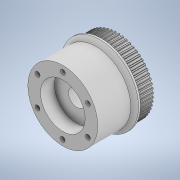
# Autodesk Inventor part: pulley_bearing_combo
Saved by Autodesk Inventor 2020.3 (Build 243373000, 373)
## iProperties
Created: 2020-11-01
Part Number: pulley_bearing_combo
Material: Generic
Document SubType Name: Modeling
Designer: Martijn
Density: 1 g/cm^3
Appearance: Default
Author: Martijn
Autodesk Inventor part; units mm, degrees
ref_plane "YZ Plane" through (0, 0, 0) normal (1, 0, 0) x (0, 1, 0)
ref_plane "XZ Plane" through (0, 0, 0) normal (0, 1, 0) x (-1, 0, 0)
ref_plane "XY Plane" through (0, 0, 0) normal (0, 0, 1) x (1, 0, 0)
sketch "Sketch1" plane through (0, 0, 0) normal (0, 0, 1) x (1, 0, 0)
  circle A0 centre (0, 0) radius 20
  circle A1 centre (0, 0) radius 11
  dimension "d0" = 40
  dimension "d1" = 22
  constraints: 2 centre point, 2 coincident
  measures "d0" diameter of A0
  measures "d1" diameter of A1
extrude "Extrusion1" add sketch "Sketch1" along normal blind 7
sketch "Sketch2" plane through (0, 0, 7) normal (0, 0, 1) x (1, 0, 0)
  circle A0 centre (0, 0) radius 4.3
  circle A1 centre (0, 0) radius 20
  circle A2 centre (0, 0) radius 20 projected
  dimension "d4" = 8.6
  constraints: 2 centre point, 2 coincident, 1 concentric
  measures "d4" diameter of A0
extrude "Extrusion2" add sketch "Sketch2" along normal blind 16
sketch "Sketch3" plane through (0, 0, 23) normal (0, 0, 1) x (1, 0, 0)
  circle A0 centre (0, 0) radius 90
  circle A1 centre (0, 0) radius 4.3
  circle A2 centre (0, 0) radius 4.3 projected
  dimension "d7" = 180
  constraints: 2 centre point, 2 coincident, 1 concentric
  measures "d7" diameter of A0
extrude "Extrusion3" add sketch "Sketch3" along normal blind 5
sketch "Sketch4" plane through (0, 0, 28) normal (0, 0, 1) x (1, 0, 0)
  circle A0 centre (0, 0) radius 20 projected
  circle A1 centre (0, 0) radius 11
  circle A2 centre (0, 0) radius 4.3 projected
  circle A3 centre (0, 0) radius 90
  circle A4 centre (0, 0) radius 90 projected
  dimension "d10" = 22
  constraints: 2 centre point, 2 coincident, 1 concentric
  measures "d10" diameter of A1
extrude "Extrusion4" add sketch "Sketch4" along normal blind 7 contours A0 | A3
sketch "Sketch5" plane through (0, 0, 0) normal (0, 0, -1) x (-1, 0, 0)
  circle A0 centre (0, 0) radius 20 projected
  line L0 (0, 0) -> (0, 20)
  arc A1 (-0.4919, 18.354) -> (0, 18.05) centre (0, 18.6) ccw
  circle A2 centre (0, 0) radius 4.3 projected
  arc A3 (-0.5869, 18.657) -> (-0.4919, 18.354) centre (0.4, 18.8) ccw
  line L1 (0.4, 18.8) -> (0, 18.8)
  line L2 (0, -98) -> (0, 98) projected
  arc A4 (-0.5869, 18.657) -> (-0.7413, 18.7854) centre (-0.7354, 18.6355) ccw
  line L3 (-1.0467, 19.9726) -> (0, 0)
  arc A5 (-0.7413, 18.7854) -> (-0.9839, 18.7742) centre (0, 0) ccw
  line L4 (-0.9839, 18.7742) -> (-1.0467, 19.9726)
  line L5 (0, 18.05) -> (0, 18.8)
  line L6 (0, 18.8) -> (0, 20)
  dimension "d14" = 0.55
  dimension "d17" = 0.4
  dimension "d18" = 0.75
  dimension "d19" = 0.15
  dimension "d20" = 3
  dimension "d22" = 18.8
  constraints: 12 end point, 10 point on circle, 5 point on line, 4 centre point, 4 collinear, 3 tangent, 1 coincident, 1 equal length, 1 perpendicular
  measures "d14" radius of A1
  measures "d17" distance of L1.start L1.end
  measures "d18" distance of L5.start L1.end
  measures "d19" radius of A4
  measures "d20" angle of L3 L0
  measures "d22" distance of L1.end L0.start
extrude "Extrusion5" cut sketch "Sketch5" against normal blind 8 contours L0 A1 A3 A4 A5 L3 A0
mirror "Mirror1" about plane through (0, 20, 0) normal (1, 0, 0) of "Extrusion5"
pattern_circular "Circular Pattern1" count 60 over 360 about axis through (0, 0, 7) along (0, 0, 1) of "Extrusion5", "Mirror1"
sketch "Sketch6" plane through (0, 0, 0) normal (0, 0, -1) x (-1, 0, 0)
  circle A0 centre (14, 0) radius 1.25
  line L0 (98, 0) -> (-98, 0) projected
  point P0 (0, 0)
  dimension "d28" = 2.5
  dimension "d29" = 14
  constraints: 1 centre point, 1 point on line
  measures "d28" diameter of A0
  measures "d29" distance of A0.centre point (0, 0)
extrude "Extrusion6" cut sketch "Sketch6" against normal blind 23
pattern_circular "Circular Pattern2" count 3 over 360 about axis through (0, 0, 7) along (0, 0, 1) of "Extrusion6"
sketch "Sketch7" plane through (0, 0, 28) normal (0, 0, 1) x (1, 0, 0)
  circle A0 centre (0, 0) radius 7.5
  dimension "d35" = 15
  constraints: 1 centre point, 1 coincident
  measures "d35" diameter of A0
extrude "Extrusion7" cut sketch "Sketch7" against normal blind 7.2
sketch "Sketch8" plane through (0, 0, 35) normal (0, 0, 1) x (1, 0, 0)
  circle A0 centre (-80, 0) radius 1.6
  circle A1 centre (-78.7846, 13.8919) radius 1.6
  circle A2 centre (-39.8478, 3.4862) radius 1.6
  circle A3 centre (0, 0) radius 4.3 projected
  line L0 (-80, 0) -> (0, 0)
  line L1 (0, 0) -> (-39.8478, 3.4862)
  line L2 (-78.7846, 13.8919) -> (0, 0)
  dimension "d38" = 10
  dimension "d39" = 5
  dimension "d40" = 3.2
  dimension "d41" = 3.2
  dimension "d42" = 3.2
  dimension "d43" = 80
  dimension "d44" = 80
  dimension "d45" = 40
  constraints: 6 end point, 3 centre point, 1 horizontal
  measures "d38" angle of L0 L2
  measures "d39" angle of L0 L1
  measures "d40" diameter of A2
  measures "d41" diameter of A0
  measures "d42" diameter of A1
  measures "d43" distance of L0.start L0.end
  measures "d44" distance of L2.start L0.end
  measures "d45" distance of L0.end L1.end
extrude "Extrusion8" cut sketch "Sketch8" against normal through all contours A0 | A1 | A2
sketch "Sketch9" plane through (0, 0, 23) normal (0, 0, 1) x (1, 0, 0)
  line L0 (-77.15, -1.6454) -> (-77.15, 1.6454)
  line L1 (-77.15, 1.6454) -> (-80, 3.2909)
  line L2 (-80, 3.2909) -> (-82.85, 1.6454)
  line L3 (-82.85, 1.6454) -> (-82.85, -1.6454)
  line L4 (-82.85, -1.6454) -> (-80, -3.2909)
  line L5 (-80, -3.2909) -> (-77.15, -1.6454)
  line L6 (-77.15, 1.6454) -> (-82.85, -1.6454)
  circle A0 centre (-80, 0) radius 1.6 projected
  circle A1 centre (-80, 0) radius 1.6
  circle A2 centre (-80, 0) radius 1.6 projected
  line L7 (-76.2636, 11.7765) -> (-75.6922, 15.0174)
  line L8 (-75.6922, 15.0174) -> (-78.2132, 17.1328)
  line L9 (-78.2132, 17.1328) -> (-81.3056, 16.0072)
  line L10 (-81.3056, 16.0072) -> (-81.8771, 12.7663)
  line L11 (-81.8771, 12.7663) -> (-79.3561, 10.651)
  line L12 (-79.3561, 10.651) -> (-76.2636, 11.7765)
  line L13 (-79.3561, 10.651) -> (-78.2132, 17.1328)
  circle A3 centre (-78.7846, 13.8919) radius 1.6 projected
  circle A4 centre (-78.7846, 13.8919) radius 1.6
  circle A5 centre (-78.7846, 13.8919) radius 1.6 projected
  line L14 (-37.152, 1.5986) -> (-40.1346, 0.2079)
  line L15 (-40.1346, 0.2079) -> (-42.8304, 2.0954)
  line L16 (-42.5435, 5.3738) -> (-39.561, 6.7646)
  line L17 (-39.561, 6.7646) -> (-36.8652, 4.877)
  line L18 (-36.8652, 4.877) -> (-42.8304, 2.0954)
  circle A6 centre (-39.8478, 3.4862) radius 1.6 projected
  circle A7 centre (-39.8478, 3.4862) radius 1.6
  line L19 (-42.8304, 2.0954) -> (-42.5435, 5.3738)
  line L20 (-37.152, 1.5986) -> (-36.8652, 4.877)
  point P0 (0, 0)
  point P1 (-78.7846, 13.8919)
  point P2 (-39.8478, 3.4862)
  dimension "d48" = 120
  dimension "d49" = 120
  dimension "d50" = 5.7
  dimension "d51" = 120
  dimension "d52" = 120
  dimension "d53" = 5.7
  dimension "d54" = 170
  dimension "d55" = 120
  dimension "d60" = 5.7
  dimension "d61" = 120
  dimension "d62" = 120
  dimension "d63" = 5
  constraints: 42 end point, 13 equal length, 6 coincident, 5 concentric, 4 parallel, 3 centre point, 3 midpoint, 1 vertical
  measures "d48" angle of L4 L3
  measures "d49" angle of L5 L4
  measures "d50" distance between parallel lines of L3 L0
  measures "d51" angle of L12 L11
  measures "d52" angle of L7 L12
  measures "d53" distance between parallel lines of L7 L10
  measures "d54" angle of L0 L7
  measures "d55" angle of L15 L14
  measures "d60" distance between parallel lines of L16 L14
  measures "d61" angle of L20 L14
  measures "d62" angle of L17 L20
  measures "d63" angle of L0 L20
extrude "Extrusion10" cut sketch "Sketch9" along normal blind 5 contours L5 L4 L6 A0 L0 | L6 A0 L3 L2 L1 | L12 L13 A3 L8 L7 | L11 L10 L9 L13 A3 | L14 L15 L18 A6 L20 | L18 A6 L19 L16 L17
pattern_circular "Circular Pattern4" count 18 over 360 about axis through (0, 0, 0) along (0, 0, 1) of "Extrusion10", "Extrusion8"
sketch "Sketch11" plane through (0, 0, 35) normal (0, 0, 1) x (1, 0, 0)
  circle A0 centre (0, 0) radius 4.3 projected
  circle A1 centre (0, 0) radius 11
  circle A2 centre (0, 0) radius 11 projected
  circle A3 centre (0, 0) radius 11 projected
  circle A4 centre (0, 0) radius 90
  circle A5 centre (0, 0) radius 90 projected
  constraints: 3 concentric, 2 centre point, 2 coincident
extrude "Extrusion12" cut sketch "Sketch11" against normal up to surface (7 mm away) contours A4
sketch "Sketch12" plane through (0, 0, 28) normal (0, 0, 1) x (1, 0, 0)
  circle A0 centre (0, 0) radius 4.3 projected
  circle A1 centre (0, 0) radius 20
  circle A2 centre (0, 0) radius 20 projected
  circle A3 centre (0, 0) radius 7.5 projected
  circle A4 centre (0, 0) radius 90
  circle A5 centre (0, 0) radius 90 projected
  constraints: 3 concentric, 2 centre point, 2 coincident
extrude "Extrusion13" cut sketch "Sketch12" against normal blind 10 contours A4
sketch "Sketch13" plane through (0, 0, 28) normal (0, 0, 1) x (1, 0, 0)
  circle A0 centre (-0.0531, -14.9999) radius 1.25
  point P0 (0, 0)
  dimension "d80" = 2.5
  dimension "d81" = 15
  constraints: 1 centre point
  measures "d80" diameter of A0
  measures "d81" distance of point (0, 0) A0.centre
extrude "Extrusion14" cut sketch "Sketch13" against normal blind 20
pattern_circular "Circular Pattern5" count 6 over 360 about axis through (0, 0, 28) along (0, 0, -1) of "Extrusion14"
sketch "Sketch14" plane through (0, 0, 28) normal (0, 0, 1) x (1, 0, 0)
  circle A0 centre (0, 0) radius 18
  circle A1 centre (0, 0) radius 20 projected
  dimension "d87" = 2
  constraints: 1 centre point, 1 coincident
  measures "d87" radial gap between concentric circles of A0 A1
extrude "Extrusion15" cut sketch "Sketch14" against normal blind 19
chamfer "Chamfer1" distance 2 angle 45 1 edges at (-18, 0, 9)
sketch "Sketch16" plane through (0, 0, 28) normal (0, 0, 1) x (1, 0, 0)
  circle A0 centre (0, 0) radius 11.5
  dimension "d93" = 23
  constraints: 1 centre point, 1 coincident
  measures "d93" diameter of A0
extrude "Extrusion16" cut sketch "Sketch16" against normal up to surface (7.2 mm away)
body "Solid1"
